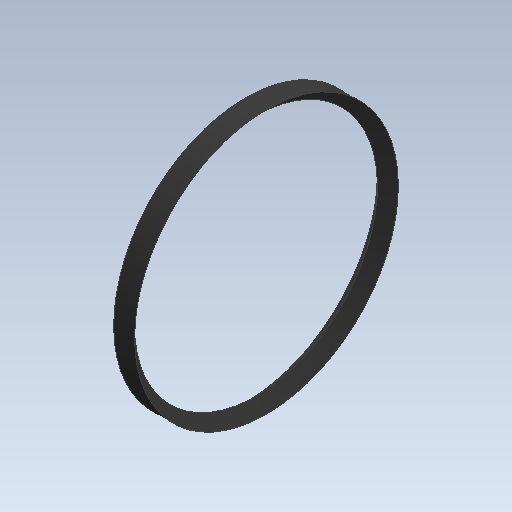
# Autodesk Inventor part: hull_seal
Saved by Autodesk Inventor 2020.2 (Build 242310000, 310)
## iProperties
Created: 2020-03-22
Part Number: hull_seal
Material: Rubber, Silicone
Document SubType Name: Modeling
Designer: agmle
Density: 1.25 g/cm^3
Appearance: Rubber - Black
Mass: 63.0208 g
Surface Area: 281.567 cm^2
Volume: 50.4166 cm^3
Author: agmle
Autodesk Inventor part; units mm, degrees
ref_plane "YZ Plane" through (0, 0, 0) normal (1, 0, 0) x (0, 1, 0)
ref_plane "XZ Plane" through (0, 0, 0) normal (0, 1, 0) x (-1, 0, 0)
ref_plane "XY Plane" through (0, 0, 0) normal (0, 0, 1) x (1, 0, 0)
sketch "Sketch1" plane through (0, 0, 0) normal (1, 0, 0) x (0, 1, 0)
  circle A0 centre (0, 0) radius 109.5375
  dimension "d0" = 219.075
  constraints: 1 centre point, 1 coincident
  measures "d0" diameter of A0
sketch "Sketch2" plane through (0, 0, 0) normal (0, 0, 1) x (1, 0, 0)
  line L0 (-8.6741, 109.5375) -> (8.6741, 109.5375)
  line L1 (8.6741, 109.5375) -> (0, 100.8634)
  line L2 (0, 100.8634) -> (-8.6741, 109.5375)
  line L3 (0, -109.5375) -> (0, 109.5375) construction
  point P0 (0, 0)
  dimension "d1" = 8.6741
  constraints: 6 end point, 2 perpendicular, 1 horizontal, 1 midpoint, 1 point on line
  measures "d1" distance from line of L1.end L0
sweep "Sweep1" add profiles "Sketch2" path "Sketch1"
equation "\"d0\" = hull_od"
equation "\"d1\" = hull_wall"
equation "\"hull_od\" = 219.075"
equation "\"hull_id\" = 201.7268"
equation "\"hull_wall\" = 8.6741"
equation "\"hull_length\" = 609.6"
equation "\"hull_spacing\" = 390.525"
equation "\"impeller_od\" = 76.2"
equation "\"impeller_clearance\" = 0.5"
equation "\"impeller_shaft_id\" = 3.175"
equation "\"impeller_shaft_od\" = 5.715"
equation "\"impeller_shaft_support\" = 3.175"
equation "\"impeller_intake_od\" = 19.05"
equation "\"impeller_vane_thick\" = 2"
equation "\"impeller_vane_inner_rad\" = 3.175"
equation "\"impeller_vane_outer_rad\" = 0.37206"
equation "\"magnet_od\" = 5.95"
equation "\"magnet_clearance\" = 0.25"
equation "\"magnet_rad\" = 0.25"
equation "\"magnet_circle_offset\" = 3.175"
equation "\"motor_shaft_od\" = 12.7"
equation "\"motor_shaft_length\" = 31.75"
equation "\"motor_shaft_key\" = 3.048"
equation "\"slab_thick\" = 34.671"
body "Solid1"
